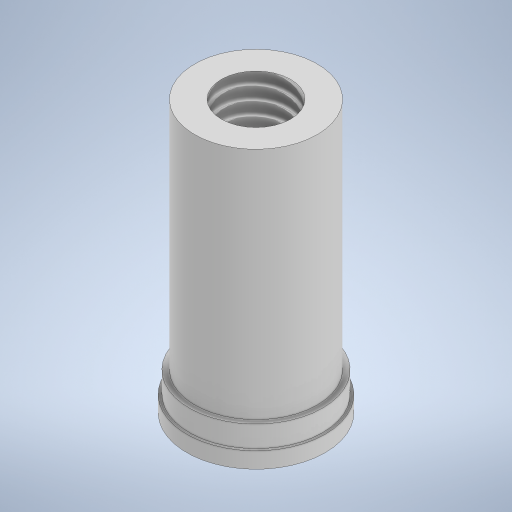
# Autodesk Inventor part: 축 볼트
Saved by Autodesk Inventor 2024 (Build 280153000, 153)
## iProperties
Created: 2023-05-25
Part Number: 축 볼트
Material: 일반
Document SubType Name: Modeling
Designer: hjcho
Density: 1 g/cm^3
Appearance: 기본값
Author: hjcho
Autodesk Inventor part; units mm, degrees
ref_plane "YZ Plane" through (0, 0, 0) normal (1, 0, 0) x (0, 1, 0)
ref_plane "XZ Plane" through (0, 0, 0) normal (0, 1, 0) x (-1, 0, 0)
ref_plane "XY Plane" through (0, 0, 0) normal (0, 0, 1) x (1, 0, 0)
sketch "스케치1" plane through (0, 0, 0) normal (0, 1, 0) x (-1, 0, 0)
  circle A0 centre (0, 0) radius 2.6
  dimension "d0" = 5.2
  constraints: 1 centre point, 1 coincident
  measures "d0" diameter of A0
extrude "돌출1" add sketch "스케치1" along normal blind 0.6
sketch "스케치2" plane through (0, 0.6, 0) normal (0, 1, 0) x (1, 0, 0)
  circle A0 centre (0, 0) radius 2.5
  dimension "d3" = 5
  constraints: 1 centre point, 1 coincident
  measures "d3" diameter of A0
extrude "돌출2" add sketch "스케치2" along normal blind 0.8
sketch "스케치3" plane through (0, 1.4, 0) normal (0, 1, 0) x (1, 0, 0)
  circle A0 centre (0, 0) radius 2.3
  dimension "d6" = 4.6
  constraints: 1 centre point, 1 coincident
  measures "d6" diameter of A0
extrude "돌출3" add sketch "스케치3" along normal blind 8.795
sketch "스케치4" plane through (0, 10.195, 0) normal (0, 1, 0) x (1, 0, 0)
  circle A0 centre (0, 0) radius 1.3
  dimension "d9" = 2.6
  constraints: 1 centre point, 1 coincident
  measures "d9" diameter of A0
extrude "돌출4" cut sketch "스케치4" against normal blind 6
thread "스레드1" size "M3x0.5" class "6H" standard "ANSI Metric M Profile" length 35
